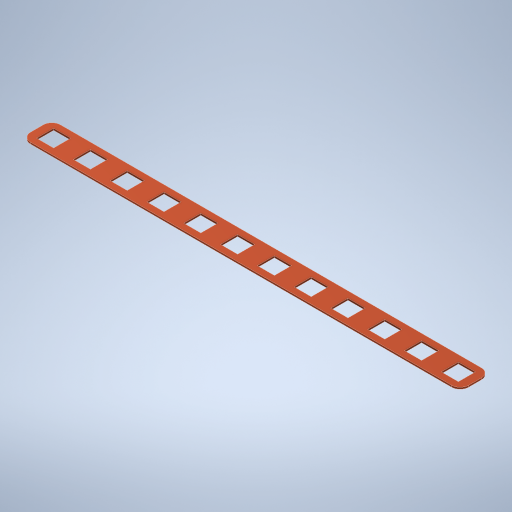
# Autodesk Inventor part: bat_contacts_v2_plate_long
Saved by Autodesk Inventor 2024 (Build 280153000, 153)
## iProperties
Created: 2025-05-07
Part Number: bat_contacts_v2_plate_long
Material: Kupfer
Document SubType Name: Modellieren
Designer: David
Density: 8.94 g/cm^3
Appearance: Kupfer - satiniert
Sheet Metal Rule: Standard_mm
Author: David
Autodesk Inventor part; units mm, degrees
ref_plane "YZ Plane" through (0, 0, 0) normal (1, 0, 0) x (0, 1, 0)
ref_plane "XZ Plane" through (0, 0, 0) normal (0, 1, 0) x (-1, 0, 0)
ref_plane "XY Plane" through (0, 0, 0) normal (0, 0, 1) x (1, 0, 0)
sketch "Skizze1" plane through (0, 0, 0) normal (0, 0, 1) x (1, 0, 0)
  line L0 (0, 0) -> (256, 0)
  line L1 (256, 0) -> (256, 17.5)
  line L2 (256, 17.5) -> (0, 17.5)
  line L3 (0, 17.5) -> (0, 0)
  line L4 (4.75, 3.75) -> (14.75, 3.75)
  line L5 (14.75, 3.75) -> (14.75, 13.75)
  line L6 (14.75, 13.75) -> (4.75, 13.75)
  line L7 (4.75, 13.75) -> (4.75, 3.75)
  line L8 (36.25, 3.75) -> (36.25, 13.75)
  line L9 (36.25, 13.75) -> (26.25, 13.75)
  line L10 (26.25, 13.75) -> (26.25, 3.75)
  line L11 (26.25, 3.75) -> (36.25, 3.75)
  line L12 (57.75, 3.75) -> (57.75, 13.75)
  line L13 (57.75, 13.75) -> (47.75, 13.75)
  line L14 (47.75, 13.75) -> (47.75, 3.75)
  line L15 (47.75, 3.75) -> (57.75, 3.75)
  line L16 (79.25, 3.75) -> (79.25, 13.75)
  line L17 (79.25, 13.75) -> (69.25, 13.75)
  line L18 (69.25, 13.75) -> (69.25, 3.75)
  line L19 (69.25, 3.75) -> (79.25, 3.75)
  line L20 (100.75, 3.75) -> (100.75, 13.75)
  line L21 (100.75, 13.75) -> (90.75, 13.75)
  line L22 (90.75, 13.75) -> (90.75, 3.75)
  line L23 (90.75, 3.75) -> (100.75, 3.75)
  line L24 (122.25, 3.75) -> (122.25, 13.75)
  line L25 (122.25, 13.75) -> (112.25, 13.75)
  line L26 (112.25, 13.75) -> (112.25, 3.75)
  line L27 (112.25, 3.75) -> (122.25, 3.75)
  line L28 (143.75, 3.75) -> (143.75, 13.75)
  line L29 (143.75, 13.75) -> (133.75, 13.75)
  line L30 (133.75, 13.75) -> (133.75, 3.75)
  line L31 (133.75, 3.75) -> (143.75, 3.75)
  line L32 (165.25, 3.75) -> (165.25, 13.75)
  line L33 (165.25, 13.75) -> (155.25, 13.75)
  line L34 (155.25, 13.75) -> (155.25, 3.75)
  line L35 (155.25, 3.75) -> (165.25, 3.75)
  line L36 (186.75, 3.75) -> (186.75, 13.75)
  line L37 (186.75, 13.75) -> (176.75, 13.75)
  line L38 (176.75, 13.75) -> (176.75, 3.75)
  line L39 (176.75, 3.75) -> (186.75, 3.75)
  line L40 (208.25, 3.75) -> (208.25, 13.75)
  line L41 (208.25, 13.75) -> (198.25, 13.75)
  line L42 (198.25, 13.75) -> (198.25, 3.75)
  line L43 (198.25, 3.75) -> (208.25, 3.75)
  line L44 (229.75, 3.75) -> (229.75, 13.75)
  line L45 (229.75, 13.75) -> (219.75, 13.75)
  line L46 (219.75, 13.75) -> (219.75, 3.75)
  line L47 (219.75, 3.75) -> (229.75, 3.75)
  line L48 (251.25, 3.75) -> (251.25, 13.75)
  line L49 (251.25, 13.75) -> (241.25, 13.75)
  line L50 (241.25, 13.75) -> (241.25, 3.75)
  line L51 (241.25, 3.75) -> (251.25, 3.75)
  point P0 (0, 8.75)
  point P1 (128, 17.5)
  point P2 (106.5, 8.75)
  point P3 (149.5, 8.75)
  point P4 (256, 8.75)
  dimension "d0" = 256
  dimension "d1" = 17.5
  dimension "d2" = 10
  dimension "d3" = 10
  dimension "d19" = 21.5
  dimension "d24" = 43
  dimension "d25" = 21.5
  constraints: 104 end point, 4 parallel, 3 horizontal, 3 midpoint, 2 horizontal alignment, 2 perpendicular, 88 other
  measures "d0" distance of L1.end L2.end
  measures "d1" distance of L2.end L0.start
  measures "d2" distance of L6.end L4.start
  measures "d3" distance of L4.start L4.end
  measures "d19" distance of L4.end L8.start
  measures "d24" distance of point (149.5, 8.75) point (106.5, 8.75)
  measures "d25" horizontal distance of point (128, 17.5) point (106.5, 8.75)
extrude "Extrusion1" add sketch "Skizze1" along normal blind 1
fillet "Rundung1" radius 5 4 edges at (256, 17.5, 0.5) (256, 0, 0.5) (0, 17.5, 0.5) (0, 0, 0.5)
sketch "Skizze2" plane through (0, 0, 1) normal (0, 0, 1) x (1, 0, 0)
  arc A0 (0, 5) -> (5, 0) centre (5, 5) ccw projected
  line L0 (5, 0) -> (251, 0) projected
  arc A1 (251, 0) -> (256, 5) centre (251, 5) ccw projected
  line L1 (256, 5) -> (256, 12.5) projected
  arc A2 (256, 12.5) -> (251, 17.5) centre (251, 12.5) ccw projected
  line L2 (251, 17.5) -> (5, 17.5) projected
  arc A3 (5, 17.5) -> (0, 12.5) centre (5, 12.5) ccw projected
  line L3 (0, 12.5) -> (0, 5) projected
  line L4 (251.25, 3.75) -> (241.25, 3.75) projected
  line L5 (241.25, 3.75) -> (241.25, 13.75) projected
  line L6 (241.25, 13.75) -> (251.25, 13.75) projected
  line L7 (251.25, 13.75) -> (251.25, 3.75) projected
  line L8 (229.75, 3.75) -> (219.75, 3.75) projected
  line L9 (219.75, 3.75) -> (219.75, 13.75) projected
  line L10 (219.75, 13.75) -> (229.75, 13.75) projected
  line L11 (229.75, 13.75) -> (229.75, 3.75) projected
  line L12 (208.25, 3.75) -> (198.25, 3.75) projected
  line L13 (198.25, 3.75) -> (198.25, 13.75) projected
  line L14 (198.25, 13.75) -> (208.25, 13.75) projected
  line L15 (208.25, 13.75) -> (208.25, 3.75) projected
  line L16 (186.75, 3.75) -> (176.75, 3.75) projected
  line L17 (176.75, 3.75) -> (176.75, 13.75) projected
  line L18 (176.75, 13.75) -> (186.75, 13.75) projected
  line L19 (186.75, 13.75) -> (186.75, 3.75) projected
  line L20 (165.25, 3.75) -> (155.25, 3.75) projected
  line L21 (155.25, 3.75) -> (155.25, 13.75) projected
  line L22 (155.25, 13.75) -> (165.25, 13.75) projected
  line L23 (165.25, 13.75) -> (165.25, 3.75) projected
  line L24 (143.75, 3.75) -> (133.75, 3.75) projected
  line L25 (133.75, 3.75) -> (133.75, 13.75) projected
  line L26 (133.75, 13.75) -> (143.75, 13.75) projected
  line L27 (143.75, 13.75) -> (143.75, 3.75) projected
  line L28 (122.25, 3.75) -> (112.25, 3.75) projected
  line L29 (112.25, 3.75) -> (112.25, 13.75) projected
  line L30 (112.25, 13.75) -> (122.25, 13.75) projected
  line L31 (122.25, 13.75) -> (122.25, 3.75) projected
  line L32 (100.75, 3.75) -> (90.75, 3.75) projected
  line L33 (90.75, 3.75) -> (90.75, 13.75) projected
  line L34 (90.75, 13.75) -> (100.75, 13.75) projected
  line L35 (100.75, 13.75) -> (100.75, 3.75) projected
  line L36 (79.25, 3.75) -> (69.25, 3.75) projected
  line L37 (69.25, 3.75) -> (69.25, 13.75) projected
  line L38 (69.25, 13.75) -> (79.25, 13.75) projected
  line L39 (79.25, 13.75) -> (79.25, 3.75) projected
  line L40 (57.75, 3.75) -> (47.75, 3.75) projected
  line L41 (47.75, 3.75) -> (47.75, 13.75) projected
  line L42 (47.75, 13.75) -> (57.75, 13.75) projected
  line L43 (57.75, 13.75) -> (57.75, 3.75) projected
  line L44 (36.25, 3.75) -> (26.25, 3.75) projected
  line L45 (26.25, 3.75) -> (26.25, 13.75) projected
  line L46 (26.25, 13.75) -> (36.25, 13.75) projected
  line L47 (36.25, 13.75) -> (36.25, 3.75) projected
  line L48 (4.75, 3.75) -> (4.75, 13.75) projected
  line L49 (4.75, 13.75) -> (14.75, 13.75) projected
  line L50 (14.75, 13.75) -> (14.75, 3.75) projected
  line L51 (14.75, 3.75) -> (4.75, 3.75) projected
  point P0 (0, 0)
equation "\"d24\" = 2 * d19"
equation "\"d25\" = 0.5 * d24"
equation "\"Biegeradius\" = Stärke"
equation "\"BreiteBiegungsfreistellung\" = Stärke"
equation "\"TiefeBiegungsfreistellung\" = 0.5 * Stärke"
equation "\"GrößeEckenfreistellung\" = 4 * Stärke"
equation "\"MinimalRest\" = 2 * Stärke"
equation "\"Übergangsradius\" = Biegeradius"
equation "\"JacobiRadiusGröße\" = Biegeradius"
equation "\"Abstandsgröße\" = Stärke"
equation "\"Stärke\" = 0.5"
